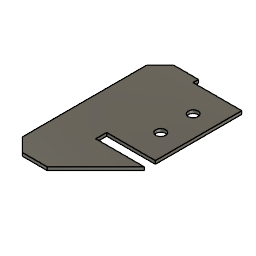
GPL H300 to 200G20_ (Autodesk Fusion 360 design; units mm, degrees)
Autodesk Fusion 360 part; units mm, degrees
sketch "スケッチ1" plane through (0, 0, 0) normal (0, 0, 1) x (1, 0, 0)
  line L0 (-9.5, 140) -> (-80.5, 140)
  line L1 (-80.5, 140) -> (-80.5, -140)
  line L2 (-80.5, -140) -> (-9.5, -140)
  line L3 (80.5, -30) -> (80.5, 130)
  line L4 (74.75, 130) -> (-80.5, -140) construction
  line L5 (-9.5, 140) -> (-9.5, 130)
  line L6 (-9.5, 130) -> (80.5, 130)
  line L7 (-80.5, -140) -> (-9.5, -140) construction
  line L8 (80.5, -50) -> (-9.5, -140)
  line L9 (80.5, -50) -> (-9.5, -50)
  line L10 (-9.5, -50) -> (-9.5, -30)
  line L11 (-9.5, -30) -> (80.5, -30)
  line L12 (-80.5, 140) -> (17.25, -30) construction
  line L13 (28.75, -50) -> (47.6429, -82.8571) construction
  dimension "d2" = 280
  dimension "d5" = 71
  dimension "d7" = 90
  dimension "d8" = 20
  constraint horizontal L0
  constraint perpendicular L0 L1
  constraint parallel L0 L2
  constraint parallel L1 L3
  constraint coincident L4 origin
  constraint coincident origin L12
  constraint vertical L5
  constraint horizontal L6
  constraint coincident L6 L4.start
  constraint perpendicular L1 L7
  constraint coincident L8 L13.end
  constraint horizontal L9
  constraint vertical L10
  constraint horizontal L11
  constraint coincident L11 L12.end
  constraint coincident L9 L13.start
  constraint collinear L12 L13
  measures "d2" distance of L0.end L1.end
  measures "d5" distance of L1.end L2.end
  measures "d7" distance of L8.start L9.end
  measures "d8" distance of L8.start L3.start
extrude "押し出し1" add sketch "スケッチ1" along normal blind 6
chamfer "面取り1" distance 25 angle 45 2 edges at (-80.5, -140, 3) (-80.5, 140, 3)
sketch "スケッチ2" plane through (0, 0, 6) normal (0, 0, 1) x (-1, 0, 0)
  line L0 (55.5, -140) -> (80.5, -115)
  line L1 (80.5, -115) -> (80.5, 115)
  line L2 (80.5, 115) -> (55.5, 140)
  line L3 (55.5, 140) -> (9.5, 140)
  line L4 (9.5, 140) -> (-80.5, 50)
  line L5 (-80.5, 50) -> (9.5, 50)
  line L6 (9.5, 50) -> (9.5, 30)
  line L7 (9.5, 30) -> (-80.5, 30)
  line L8 (-80.5, 30) -> (-80.5, -130)
  line L9 (-80.5, -130) -> (9.5, -130)
  line L10 (9.5, -130) -> (9.5, -140)
  line L11 (9.5, -140) -> (55.5, -140)
  line L12 (-80.5, -130) -> (-40.5, -130) construction
  line L13 (-40.5, -130) -> (-40.5, -80) construction
  line L14 (-40.5, -80) -> (-80.5, -80) construction
  line L15 (-80.5, -80) -> (-80.5, -130) construction
  line L16 (-40.5, -80) -> (-40.5, -20) construction
  point P0 (-40.5, -80)
  point P1 (-40.5, -20)
  dimension "d12" = 40
  dimension "d13" = 50
  dimension "d14" = 60
  constraint horizontal L12
  constraint vertical L13
  constraint horizontal L14
  constraint vertical L15
  constraint coincident L8.end L9.start
  constraint perpendicular L14 L16
  constraint coincident P0 L13.end
  constraint coincident P1 L16.end
  measures "d12" distance of L8.end L12.end
  measures "d13" distance of L8.end L14.end
  measures "d14" distance of P0 P1
hole "穴1" at (40.5, 80, 6) at (40.5, 20, 6) direction (0, 0, -1) diameter 18 end through all
equation "d5 = 25 mm + 46 mm"
